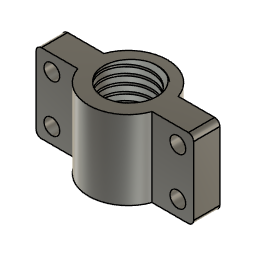
Moving_Nut_ver4 v3 (Autodesk Fusion 360 design; units mm, degrees)
Autodesk Fusion 360 part; units mm, degrees
note: some values were not read from the file. Set by a fixed rule: which sketch regions a step uses.
sketch "스케치1" plane through (0, 0, 0) normal (0, 0, 1) x (1, 0, 0)
  circle A0 centre (0, 0) radius 5.5
  line L0 (15, 2.5) -> (7.0711, 2.5)
  line L1 (7.0711, -2.5) -> (15, -2.5)
  line L2 (15, -2.5) -> (15, 2.5)
  line L3 (15, 2.5) -> (0, -2.5) construction
  line L4 (0, 2.5) -> (15, -2.5) construction
  line L5 (-7.0711, 2.5) -> (-15, 2.5)
  line L6 (-15, 2.5) -> (-15, -2.5)
  line L7 (-15, -2.5) -> (-7.0711, -2.5)
  line L8 (0, 2.5) -> (-15, -2.5) construction
  line L9 (-15, 2.5) -> (0, -2.5) construction
  arc A1 (7.0711, 2.5) -> (-7.0711, 2.5) centre (0, 0) ccw
  arc A2 (-7.0711, -2.5) -> (7.0711, -2.5) centre (0, 0) ccw
  dimension "d15" = 11
  dimension "d16" = 15
  dimension "d17" = 15
  dimension "d18" = 5
  dimension "d19" = 15
  dimension "d20" = 5
  constraint coincident A0.centre A1.centre
  constraint concentric A0 A1
  constraint horizontal L0
  constraint parallel L0 L1
  constraint horizontal L5
  constraint perpendicular L5 L6
  constraint parallel L5 L7
  constraint coincident L7.end A1
  constraint concentric A1 A2
  measures "d15" diameter of A0
  measures "d16" diameter of A1
  measures "d17" distance of L3.end L1.end
  measures "d18" distance of L4.start L3.end
  measures "d19" distance of L6.end L3.end
  measures "d20" distance of L5.end L6.end
extrude "돌출1" add sketch "스케치1" along normal blind 15
thread "나사산1" "ISO Metric profile 11.0 M11x1.5 6H" major diameter 11.1933 minor diameter 9.5262 pitch 1.5 angle 60 modelled right hand crest width 0.4125 on face at (5.4727, -0.5476, 10) crest through (4.7631, 0, 0.375)
sketch "스케치2" plane through (0, 2.5, 0) normal (0, 1, 0) x (-1, 0, 0)
  line L0 (-15, 0) -> (-7.0711, 0)
  line L1 (-7.0711, 0) -> (-7.0711, 15)
  line L2 (-7.0711, 15) -> (-15, 15)
  line L3 (-15, 15) -> (-15, 0)
  line L4 (-12, 22) -> (-12, -5)
  line L5 (12, 22) -> (12, -5)
  line L6 (15, 0) -> (15, 15)
  line L7 (-19, 12) -> (20.3222, 12)
  line L8 (-18, 3) -> (20.4544, 3)
  circle A0 centre (-12, 12) radius 1.5
  circle A1 centre (-12, 3) radius 1.5
  circle A2 centre (12, 3) radius 1.5
  circle A3 centre (12, 12) radius 1.5
  dimension "d25" = 3
  dimension "d26" = 3
  dimension "d27" = 3
  dimension "d28" = 3
  dimension "d29" = 3
  dimension "d30" = 3
  dimension "d31" = 3
  dimension "d32" = 3
  constraint vertical L4
  constraint vertical L5
  constraint perpendicular L6 L7
  constraint perpendicular L6 L8
  constraint coincident L4 A0.centre
  constraint coincident L7 A0.centre
  constraint coincident L4 A1.centre
  constraint coincident L8 A1.centre
  constraint coincident L8 A2.centre
  constraint coincident L5 A2.centre
  constraint coincident L7 A3.centre
  constraint coincident L5 A3.centre
  measures "d25" distance of L3 L4
  measures "d26" distance of L5 L6
  measures "d27" distance of L0 L8
  measures "d28" distance of L2 L7
  measures "d29" diameter of A0
  measures "d30" diameter of A1
  measures "d31" diameter of A2
  measures "d32" diameter of A3
extrude "돌출2" cut sketch "스케치2" against normal blind 5 contours L4 L8 A1 | L4 L8 A1 | L4 L8 A1 | L4 L8 A1 | L4 L7 A0 | L4 L7 A0 | L5 L8 A2 | L5 L8 A2 | L4 L7 A0 | L4 L7 A0 | L5 L7 A3 | L5 L7 A3 | L5 L8 A2 | L5 L8 A2 | L5 L7 A3 | L5 L7 A3
fillet "필렛1" radius 1 4 edges at (15, 0, 15) (-15, 0, 15) (-15, 0, 0) (15, 0, 0)
